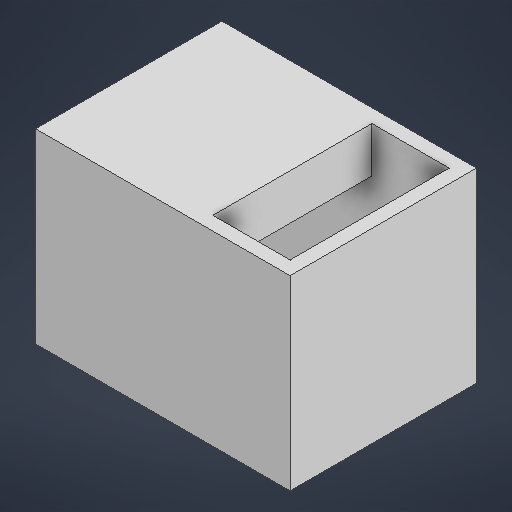
# Autodesk Inventor part: Part6
Saved by Autodesk Inventor 2026.2 (Build 302298000, 298)
## iProperties
Created: 2026-02-23
Part Number: Part6
Material: Generic
Document SubType Name: Modeling
Designer: danda
Density: 1 g/cm^3
Appearance: Default
Author: danda
Autodesk Inventor part; units mm, degrees
ref_plane "YZ Plane" through (0, 0, 0) normal (1, 0, 0) x (0, 1, 0)
ref_plane "XZ Plane" through (0, 0, 0) normal (0, 1, 0) x (-1, 0, 0)
ref_plane "XY Plane" through (0, 0, 0) normal (0, 0, 1) x (1, 0, 0)
sketch "Sketch1" plane through (0, 0, 0) normal (0, 0, 1) x (1, 0, 0)
  line L0 (6.1879, 20.8703) -> (36.1879, 20.8703)
  line L1 (36.1879, -14.1297) -> (6.1879, -14.1297)
  line L2 (39.1879, 23.8703) -> (3.1879, 23.8703)
  line L3 (3.1879, -17.1297) -> (39.1879, -17.1297)
  line L4 (56.1879, 23.8703) -> (59.1879, 23.8703)
  line L5 (59.1879, 23.8703) -> (59.1879, -17.1297)
  line L6 (59.1879, -17.1297) -> (39.1879, -17.1297)
  line L7 (56.1879, 20.8703) -> (56.1879, -14.1297)
  line L8 (56.1879, -14.1297) -> (39.1879, -14.1297)
  line L9 (36.1879, 20.8703) -> (36.1879, 13.8703)
  line L10 (36.1879, 13.8703) -> (39.1879, 13.8703)
  line L11 (36.1879, -14.1297) -> (36.1879, -7.1297)
  line L12 (36.1879, -7.1297) -> (39.1879, -7.1297)
  line L13 (36.1879, 20.8703) -> (36.1879, 13.8703)
  line L14 (36.1879, -7.1297) -> (36.1879, -14.1297)
  line L15 (39.1879, -14.1297) -> (39.1879, -7.1297)
  line L16 (39.1879, 13.8703) -> (39.1879, 20.8703)
  line L17 (3.1879, 23.8703) -> (3.1879, 20.8703)
  line L18 (3.1879, -14.1297) -> (3.1879, -17.1297)
  line L19 (6.1879, 20.8703) -> (3.1879, 20.8703)
  line L20 (6.1879, -14.1297) -> (3.1879, -14.1297)
  line L21 (39.1879, 20.8703) -> (39.1879, 23.8703)
  line L22 (56.1879, 20.8703) -> (56.1879, 23.8703)
  point P0 (0, 0)
  dimension "d1" = 35
  dimension "d2" = 3
  dimension "d3" = 20
  dimension "d5" = 7
  dimension "d6" = 7
  dimension "d7" = 30
  constraints: 46 end point, 10 perpendicular, 7 parallel, 3 horizontal, 2 point on line, 1 collinear, 1 vertical, 1 other
  measures "d1" distance of L0.end L1.start
  measures "d2" distance between parallel lines of L0 L2
  measures "d3" distance of L2.start L4.end
  measures "d5" distance of L0.end L9.end
  measures "d6" distance of L1.start L11.end
  measures "d7" distance of L1.end L1.start
extrude "Extrusion1" add sketch "Sketch1" along normal mid plane 35
sketch "Sketch2" plane through (0, 0, -17.5) normal (0, 0, -1) x (-1, 0, 0)
  line L0 (-59.1879, 23.8703) -> (-3.1879, 23.8703) projected
  line L1 (-3.1879, -17.1297) -> (-59.1879, -17.1297) projected
  line L2 (-59.1879, 23.8703) -> (-3.1879, 23.8703)
  line L3 (-3.1879, 23.8703) -> (-3.1879, -17.1297)
  line L4 (-3.1879, -17.1297) -> (-59.1879, -17.1297)
  line L5 (-59.1879, -17.1297) -> (-59.1879, 23.8703)
  point P0 (0, 0)
  constraints: 8 end point, 2 parallel, 1 horizontal, 1 perpendicular
extrude "Extrusion3" add sketch "Sketch2" along normal blind 3
sketch "Sketch3" plane through (0, 0, 17.5) normal (0, 0, 1) x (1, 0, 0)
  line L0 (3.1879, 23.8703) -> (59.1879, 23.8703) projected
  line L1 (59.1879, -17.1297) -> (3.1879, -17.1297) projected
  line L2 (3.1879, 23.8703) -> (59.1879, 23.8703)
  line L3 (59.1879, 23.8703) -> (59.1879, -17.1297)
  line L4 (59.1879, -17.1297) -> (3.1879, -17.1297)
  line L5 (3.1879, -17.1297) -> (3.1879, 23.8703)
  point P0 (0, 0)
  constraints: 8 end point, 2 parallel, 1 horizontal, 1 perpendicular
extrude "Extrusion4" add sketch "Sketch3" along normal blind 3
sketch "Sketch4" plane through (3.1879, -14.1297, -17.5) normal (0, 1, 0) x (1, 0, 0)
  line L0 (56, 3) -> (0, 3) projected
  line L1 (0, 3) -> (56, 3)
  line L2 (0, -38) -> (56, -38) projected
  line L3 (56, 3) -> (56, -38)
  line L4 (33, 0) -> (33, -35) projected
  circle A0 centre (33, -17.5) radius 4
  point P0 (-3.1879, -17.5)
  dimension "d18" = 8
  constraints: 4 end point, 1 centre point, 1 collinear, 1 midpoint, 1 perpendicular
  measures "d18" diameter of A0
extrude "Extrusion5" cut sketch "Sketch4" along normal mid plane 15
body "Solid1"
